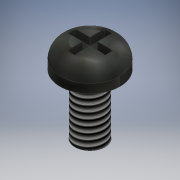
# Autodesk Inventor part: M2 Screw
Saved by Autodesk Inventor 2018 (Build 220112000, 112)
## iProperties
Created: 2018-05-10
Part Number: M2 Screw
Material: Steel
Document SubType Name: Modeling
Designer: mtsti
Density: 7.85 g/cm^3
Appearance: Plate
Author: mtsti
Autodesk Inventor part; units mm, degrees
ref_plane "YZ Plane" through (0, 0, 0) normal (1, 0, 0) x (0, 1, 0)
ref_plane "XZ Plane" through (0, 0, 0) normal (0, 1, 0) x (-1, 0, 0)
ref_plane "XY Plane" through (0, 0, 0) normal (0, 0, 1) x (1, 0, 0)
sketch "Sketch1" plane through (0, 0, 0) normal (0, 0, 1) x (1, 0, 0)
  circle A0 centre (0, 0) radius 1
  dimension "d0" = 2
  constraints: 1 centre point, 1 coincident
  measures "d0" diameter of A0
extrude "Extrusion1" add sketch "Sketch1" along normal blind 4
sketch "Sketch2" plane through (0, 0, 4) normal (0, 0, 1) x (1, 0, 0)
  circle A0 centre (0, 0) radius 2
  dimension "d3" = 4
  constraints: 1 centre point, 1 coincident
  measures "d3" diameter of A0
extrude "Extrusion2" add sketch "Sketch2" along normal blind 1.6
thread "Thread1" size "M2x0.4" class "6g" standard "ANSI Metric M Profile" full length
fillet "Fillet1" radius 1 1 edges at (-2, 0, 5.6)
sketch "Sketch3" plane through (0, 0, 5.6) normal (0, 0, 1) x (1, 0, 0)
  line L0 (-0.25, 1.25) -> (0.25, 1.25)
  line L1 (0.25, 1.25) -> (0.25, -1.25)
  line L2 (0.25, -1.25) -> (-0.25, -1.25)
  line L3 (-0.25, -1.25) -> (-0.25, 1.25)
  line L4 (-1.25, 0.25) -> (1.25, 0.25)
  line L5 (1.25, 0.25) -> (1.25, -0.25)
  line L6 (1.25, -0.25) -> (-1.25, -0.25)
  line L7 (-1.25, -0.25) -> (-1.25, 0.25)
  point P0 (0, 0)
  dimension "d9" = 0.5
  dimension "d10" = 2.5
  dimension "d11" = 2.5
  dimension "d12" = 0.5
  dimension "d13" = 0.25
  dimension "d14" = 1.25
  dimension "d15" = 0.25
  dimension "d16" = 1.25
  constraints: 16 end point, 4 parallel, 2 horizontal, 2 perpendicular
  measures "d9" distance of L1.end L2.end
  measures "d10" distance of L0.end L1.end
  measures "d11" distance of L5.end L6.end
  measures "d12" distance of L4.end L5.end
  measures "d13" distance from line of point (0, 0) L3
  measures "d14" distance from line of point (0, 0) L0
  measures "d15" distance from line of L4 point (0, 0)
  measures "d16" distance from line of point (0, 0) L7
extrude "Extrusion3" cut sketch "Sketch3" against normal blind 0.5
body "Solid1"
